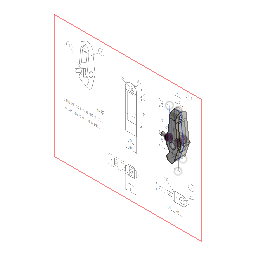
실기 (Autodesk Fusion 360 design; units mm, degrees)
Autodesk Fusion 360 part; units mm, degrees
note: some values were not read from the file. Set by a fixed rule: which sketch regions a step uses.
sketch "Sketch1" plane through (0, 0, 0) normal (0, 1, 0) x (1, 0, 0)
  circle A0 centre (0, 0) radius 5
  line L0 (0, 0) -> (-14, 0)
  line L1 (-14, 0) -> (-14, -38)
  line L2 (-14, -38) -> (-14, -45)
  line L3 (-14, 0) -> (-14, 19)
  line L4 (-14, 19) -> (8, 19)
  line L5 (0, 0) -> (0, 40)
  line L6 (0, 19) -> (-3, 19)
  line L7 (0, 0) -> (9, 0)
  line L8 (8.5622, 2.773) -> (2.7081, 20.8486)
  line L9 (0, 0) -> (0, -45)
  line L10 (-5, -45) -> (5, -45)
  line L11 (-5, -45) -> (-5, -33)
  line L12 (5, -45) -> (5, -33)
  line L13 (-5, -33) -> (-8.9324, -1.1012)
  line L14 (5, -33) -> (8.9324, -1.1012)
  arc A1 (-6.6867, 6.024) -> (-7.0709, 14.5923) centre (-11.0709, 10.1202) ccw
  arc A2 (3, 19) -> (-7, 14.5279) centre (-3, 19) ccw
  arc A3 (-6.5986, 6.1204) -> (-8.9324, -1.1012) centre (0, 0) ccw
  arc A4 (8.9324, -1.1012) -> (8.5622, 2.773) centre (0, 0) ccw
  dimension "d1" = 10
  dimension "d2" = 7
  dimension "d3" = 38
  dimension "d4" = 19
  dimension "d5" = 12
  dimension "d8" = 10
  dimension "d9" = 12
  dimension "d10" = 12
  constraint coincident A0.centre L0.start
  constraint horizontal L0
  constraint perpendicular L0 L1
  constraint parallel L1 L2
  constraint perpendicular L0 L3
  constraint perpendicular L3 L4
  constraint perpendicular L0 L5
  constraint coincident L5 L6.start
  constraint coincident L4 L6.start
  constraint midpoint L4 L6.end
  constraint coincident L6.end A2.centre
  constraint coincident L7.end A3
  constraint perpendicular L5 L7
  constraint coincident L8.end A2
  constraint tangent L8 A2
  constraint tangent L8 A3
  constraint parallel L2 L9
  constraint perpendicular L10 L11
  constraint perpendicular L10 L12
  constraint tangent L13 A3
  constraint coincident L14.end A3
  constraint tangent L14 A3
  constraint coincident A1.start A3
  constraint coincident A1.end A2
  constraint coincident A1 A3.start
  constraint coincident A1 A2.end
  constraint coincident L4 A2.start
  constraint concentric A3 A4
  measures "d1" diameter of A0
  measures "d2" distance of L1.end L2.end
  measures "d3" distance of L0.end L1.end
  measures "d4" distance of L0.end L3.end
  measures "d5" diameter of A2
  measures "d8" distance of L10.start L10.end
  measures "d9" distance of L10.start L11.end
  measures "d10" distance of L10.end L12.end
extrude "Extrude1" add sketch "Sketch1" along normal mid plane 18 contours A0 L7 L9 L10 L12 L14 A4 | A0 L4 L5 L7 L8 A4 | A0 L0 L4 L5 L6 A1 A2 A3 | A0 L0 L9 L10 L11 L13 A3 | L4 L5 A2 | L4 L5 L6 A2 makes body 1
sketch "Sketch2" plane through (-5, 0, 0) normal (-1, 0, 0) x (0, -1, 0)
  line L0 (9, 45) -> (-9, 45)
  line L1 (-9, 45) -> (-9, 33)
  line L2 (-9, 33) -> (9, 33)
  line L3 (9, 33) -> (9, 45)
  line L4 (0, 33) -> (0, 31)
  line L5 (0, 31) -> (-5, 31)
  line L6 (-5, 31) -> (-5, -9)
  line L7 (-5, -9) -> (5, -9)
  line L8 (5, -9) -> (5, 31)
  line L9 (5, 31) -> (0, 31)
  line L10 (0, 45) -> (0, 38)
  circle A0 centre (0, 38) radius 3
  dimension "d14" = 2
  dimension "d15" = 5
  dimension "d16" = 40
  dimension "d17" = 10
  dimension "d20" = 7
  dimension "d21" = 6
  constraint midpoint L2 L4.start
  constraint perpendicular L2 L4
  constraint perpendicular L4 L5
  constraint perpendicular L5 L6
  constraint perpendicular L6 L7
  constraint perpendicular L5 L8
  constraint perpendicular L4 L9
  constraint midpoint L0 L10.start
  constraint perpendicular L0 L10
  constraint coincident L10.end A0.centre
  measures "d14" distance of L4.start L4.end
  measures "d15" distance of L4.end L5.end
  measures "d16" distance of L5.end L6.end
  measures "d17" distance of L6.end L7.end
  measures "d20" distance of L10.start L10.end
  measures "d21" diameter of A0
extrude "Extrude3" cut sketch "Sketch2" against normal blind 36.418 contours A0 bodies 1
extrude "Extrude2" cut sketch "Sketch2" along normal mid plane 75.984 contours L5 L6 L7 L8 L9 bodies 1
sketch "Sketch3" plane through (0, 9, 0) normal (0, 1, 0) x (-1, 0, 0)
  circle A0 centre (0, 0) radius 5
  line L0 (5, 45) -> (-5, 45)
  line L1 (-5, 45) -> (-5, 33)
  line L2 (-5, 33) -> (-8.9324, 1.1012)
  arc A1 (-8.9324, 1.1012) -> (-8.5622, -2.773) centre (0, 0) ccw
  line L3 (-8.5622, -2.773) -> (-3.3068, -19)
  line L4 (-3.3068, -19) -> (-3, -19)
  arc A2 (-3, -19) -> (7.0709, -14.5923) centre (3, -19) ccw
  arc A3 (6.6867, -6.024) -> (7.0709, -14.5923) centre (11.0709, -10.1202) ccw
  arc A4 (6.6867, -6.024) -> (8.9324, 1.1012) centre (0, 0) ccw
  line L5 (8.9324, 1.1012) -> (5, 33)
  line L6 (5, 33) -> (5, 45)
  circle A5 centre (0, 0) radius 4.5
  circle A6 centre (0, 0) radius 7.5
  line L7 (0, 0) -> (0, -7.5)
  line L8 (0, -7.5) -> (15, -7.5)
  line L9 (0, 0) -> (0, 7.5)
  line L10 (0, 7.5) -> (15, 7.5)
  line L11 (15, 7.5) -> (15, -7.5)
  dimension "d24" = 9
  dimension "d25" = 15
  dimension "d26" = 15
  dimension "d27" = 15
  constraint concentric A0 A5
  constraint coincident A0.centre A1.centre
  constraint coincident A6 L7.end
  constraint vertical L7
  constraint perpendicular L7 L8
  constraint coincident A6 L9.end
  constraint parallel L7 L9
  constraint perpendicular L9 L10
  measures "d24" diameter of A5
  measures "d25" diameter of A6
  measures "d26" distance of L7.end L8.end
  measures "d27" distance of L9.end L10.end
extrude "Extrude4" add sketch "Sketch3" against normal blind 4 separate body contours A5 L7 L9 | A5 L7 L9 makes body 2
extrude "Extrude5" add sketch "Sketch3" against normal blind 10 from surface at -4 separate body contours A0 A5 L7 L9 | A0 A6 L7 L9 | A0 A5 L7 L9 | A0 A6 L7 L9 | A5 L7 L9 | A5 L7 L9 | A3 A4 L5 A6 L8 L10 | A3 A4 L5 L8 L10 L11 makes body 3
extrude "Extrude6" add sketch "Sketch3" against normal blind 4 from surface at -14 contours A5 L7 L9 | A5 L7 L9 bodies 3
combine "Combine1" operation add target body 3 tool bodies 2
chamfer "Chamfer1" distance 2 angle 45 4 edges at (-15, 0, 7.5) (-15, 5, 0) (-15, -5, 0) (-15, 0, -7.5) on bodies 3
sketch "Sketch4" plane through (-15, 0, 0) normal (-1, 0, 0) x (0, -1, 0)
  line L0 (-3, -5.5) -> (3, -5.5)
  line L1 (3, -5.5) -> (3, 5.5)
  line L2 (3, 5.5) -> (-3, 5.5)
  line L3 (-3, 5.5) -> (-3, -5.5)
  circle A0 centre (0, 0) radius 2.5
  dimension "d37" = 5
  constraint coincident A0.centre origin
  measures "d37" diameter of A0
extrude "Extrude7" add sketch "Sketch4" along normal blind 10 contours A0 bodies 3
fillet "Fillet1" radius 8 2 edges at (0, 9, 45) (0, -9, 45) on bodies 1
